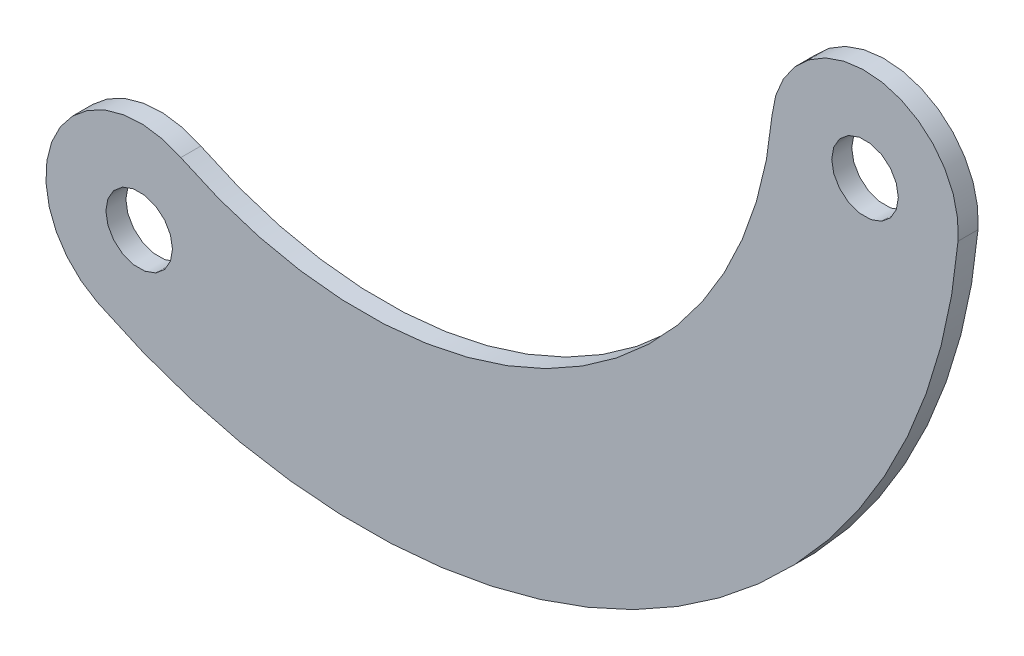
# Autodesk Inventor part: Barra estabilizadora de ascenso
Saved by Autodesk Inventor 2019 (Build 230136000, 136)
## iProperties
Created: 2020-02-06
Part Number: Barra estabilizadora de ascenso
Material: Generic
Document SubType Name: Modeling
Designer: Juan Carlos Botero
Density: 1 g/cm^3
Appearance: Default
Author: Juan Carlos Botero
Autodesk Inventor part; units mm, degrees
ref_plane "YZ Plane" through (0, 0, 0) normal (1, 0, 0) x (0, 1, 0)
ref_plane "XZ Plane" through (0, 0, 0) normal (0, 1, 0) x (-1, 0, 0)
ref_plane "XY Plane" through (0, 0, 0) normal (0, 0, 1) x (1, 0, 0)
sketch "Sketch1" plane through (0, 0, 0) normal (0, 0, 1) x (1, 0, 0)
  circle A0 centre (0, 0) radius 10
  arc A1 (-217.9737, -122.4233) -> (0, 0) centre (-150.5791, 12.843) ccw construction
  arc A2 (-230.4735, -147.5114) -> (27.9282, -2.382) centre (-150.5791, 12.843) ccw
  arc A3 (-205.4739, -97.3352) -> (-27.9282, 2.382) centre (-150.5791, 12.843) ccw
  arc A4 (-205.4739, -97.3352) -> (-230.4735, -147.5114) centre (-217.9737, -122.4233) ccw
  arc A5 (27.9282, -2.382) -> (-27.9282, 2.382) centre (0, 0) ccw
  circle A6 centre (-217.9737, -122.4233) radius 10
  dimension "d1" = 20
  dimension "d3" = 250
  constraints: 10 point on circle, 7 centre point, 4 tangent, 2 coincident, 1 equal radius
  measures "d1" diameter of A0
  measures "d3" distance of point (0, 0) A1.start
extrude "Extrusion1" add sketch "Sketch1" along normal blind 6
body "Solid1"
